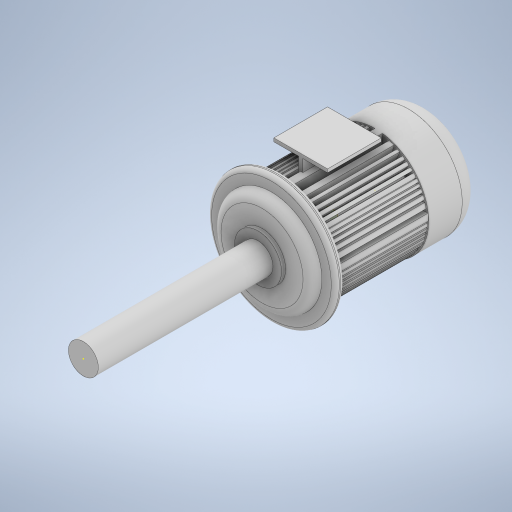
# Autodesk Inventor part: chanti eg
Saved by Autodesk Inventor 2023 (Build 270158000, 158)
## iProperties
Created: 2023-11-02
Part Number: chanti eg
Material: Generic
Document SubType Name: Modeling
Designer: chanti
Density: 1 g/cm^3
Appearance: Default
Author: chanti
Autodesk Inventor part; units mm, degrees
ref_plane "YZ Plane" through (0, 0, 0) normal (1, 0, 0) x (0, 1, 0)
ref_plane "XZ Plane" through (0, 0, 0) normal (0, 1, 0) x (-1, 0, 0)
ref_plane "XY Plane" through (0, 0, 0) normal (0, 0, 1) x (1, 0, 0)
sketch "Sketch1" plane through (0, 0, 0) normal (0, 0, 1) x (1, 0, 0)
  circle A0 centre (0, 0) radius 40
  dimension "d0" = 80
  constraints: 1 centre point, 1 coincident
  measures "d0" diameter of A0
extrude "Extrusion1" add sketch "Sketch1" along normal blind 40
sketch "Sketch2" plane through (0, 0, 40) normal (0, 0, 1) x (1, 0, 0)
  circle A0 centre (0, 0) radius 30
  dimension "d3" = 60
  constraints: 1 centre point, 1 coincident
  measures "d3" diameter of A0
sketch "Sketch3" plane through (0, 0, 40) normal (0, 0, 1) x (1, 0, 0)
  line L0 (-0.020624, 29.697668) -> (-0.020624, 39.999995)
  circle A0 centre (0, 0) radius 40
  line L1 (5.634227, 39.601206) -> (5.191892, 29.470084)
  line L2 (5.191892, 29.470084) -> (-0.020624, 29.697668)
  dimension "d4" = 2.5
  constraints: 6 end point, 2 point on circle, 1 perpendicular, 1 vertical
  measures "d4" angle of L0 L1
extrude "Extrusion2" add sketch "Sketch3" along normal blind 70 contours L0 A0 L1 L2 picked at (2.975845, 32.996997)
sketch "Sketch4" plane through (0, 0, 40) normal (0, 0, 1) x (1, 0, 0)
  circle A0 centre (0, 0) radius 40
  line L0 (0, -40) -> (0, -30.033316)
  line L1 (0, -30.033316) -> (2.293817, -30.033316)
  line L2 (2.293817, -30.033316) -> (2.710552, -40)
  line L3 (2.710552, -40) -> (0, -40)
  point P0 (0, -35.016658)
  dimension "d7" = 2.5
  constraints: 8 end point, 2 perpendicular, 1 midpoint, 1 vertical, 1 vertical alignment, 1 other
  measures "d7" distance from line of point (0, -35.017) L2
extrude "Extrusion3" add sketch "Sketch4" along normal blind 70 contours L0 L1 L2 A0 | A0 L2 L3 picked at (1.065557, -33.352147)
sketch "Sketch5" plane through (0, 0, 40) normal (0, 0, 1) x (1, 0, 0)
  circle A0 centre (0, 0) radius 40
  line L0 (6.760588, -39.424541) -> (5.721207, -29.502254)
  line L1 (5.721207, -29.502254) -> (7.131952, -29.354476)
  line L2 (7.131952, -29.354476) -> (10.234211, -38.207292)
  line L3 (10.234211, -38.207292) -> (6.760588, -39.424541)
  point P0 (8.683082, -33.780884)
  dimension "d10" = 2.5
  constraints: 8 end point, 2 perpendicular, 1 midpoint, 2 other
  measures "d10" distance from line of point (8.683, -33.781) L0
extrude "Extrusion4" add sketch "Sketch5" along normal blind 70 contours L0 L1 L2 L3
sketch "Sketch6" plane through (0, 0, 40) normal (0, 0, 1) x (1, 0, 0)
  line L0 (-11.207509, 27.841165) -> (-12.326876, 38.053227)
  circle A0 centre (0, 0) radius 40
  line L1 (-9.924989, 39.08492) -> (-8.805622, 28.872858)
  line L2 (-8.805622, 28.872858) -> (-11.207509, 27.841165)
  line L3 (-9.924989, 39.08492) -> (-12.326876, 38.053227)
  line L4 (-17.739765, 24.864744) -> (-18.904942, 35.49473)
  line L5 (-18.904942, 35.49473) -> (-21.743257, 32.947196)
  line L6 (-21.743257, 32.947196) -> (-19.480863, 23.302019)
  line L7 (-19.480863, 23.302019) -> (-17.739765, 24.864744)
  point P0 (-20.61206, 28.124608)
  point P1 (-9.365305, 33.978889)
  dimension "d13" = 2.5
  dimension "d14" = 2.5
  constraints: 16 end point, 4 parallel, 2 midpoint, 2 other
  measures "d13" distance from line of L4 point (-20.612, 28.125)
  measures "d14" distance from line of point (-9.365, 33.979) L0
extrude "Extrusion5" add sketch "Sketch6" along normal blind 70 contours L4 L7 L6 L5 A0 | A0 L5 L4
sketch "Sketch7" plane through (0, 0, 40) normal (0, 0, 1) x (1, 0, 0)
  point P0 (0, 0)
sketch "Sketch8" plane through (0, 0, 40) normal (0, 0, 1) x (1, 0, 0)
  line L0 (30.442143, 0) -> (39.650787, 0)
  line L1 (39.650787, 0) -> (39.650787, 5.274002)
  arc A0 (6.760588, -39.424541) -> (5.634227, 39.601206) centre (0, 0) ccw
  line L2 (30.442143, 4.39287) -> (30.442143, 0)
  line L3 (30.442143, 4.39287) -> (39.650787, 5.274002)
  constraints: 8 end point, 1 horizontal, 1 parallel, 1 perpendicular, 1 point on circle
extrude "Extrusion6" add sketch "Sketch8" along normal blind 70
sketch "Sketch9" plane through (0, 0, 40) normal (0, 0, 1) x (1, 0, 0)
  line L0 (10.675749, 37.596929) -> (8.268351, 29.06161)
  line L1 (8.268351, 29.06161) -> (12.000604, 28.008924)
  line L2 (12.000604, 28.008924) -> (14.408001, 36.544243)
  line L3 (14.408001, 36.544243) -> (10.675749, 37.596929)
  point P0 (0, 0)
  constraints: 8 end point, 3 perpendicular
extrude "Extrusion7" add sketch "Sketch9" along normal blind 70
sketch "Sketch10" plane through (0, 0, 40) normal (0, 0, 1) x (1, 0, 0)
  line L0 (13.617247, 27.55159) -> (16.676639, 35.171207)
  line L1 (16.676639, 35.171207) -> (18.671094, 34.300788)
  line L2 (18.671094, 34.300788) -> (15.388296, 26.77867)
  line L3 (15.388296, 26.77867) -> (13.617247, 27.55159)
  point P0 (0, 0)
  constraints: 8 end point, 2 perpendicular
extrude "Extrusion8" add sketch "Sketch10" along normal blind 70
sketch "Sketch11" plane through (0, 0, 40) normal (0, 0, 1) x (1, 0, 0)
  line L0 (16.809785, 25.989212) -> (20.82419, 32.823259)
  line L1 (20.82419, 32.823259) -> (22.496859, 31.15059)
  line L2 (22.496859, 31.15059) -> (18.182558, 25.182829)
  arc A0 (18.182558, 25.182829) -> (16.809785, 25.989212) centre (13.257658, 18.370456) ccw
  point P0 (0, 0)
  constraints: 6 end point, 2 point on circle, 1 centre point, 1 point on line
extrude "Extrusion9" add sketch "Sketch11" along normal blind 70
sketch "Sketch12" plane through (0, 0, 40) normal (0, 0, 1) x (1, 0, 0)
  line L0 (19.103485, 24.559546) -> (23.864166, 30.764478)
  line L1 (23.864166, 30.764478) -> (25.415399, 28.785319)
  line L2 (25.415399, 28.785319) -> (21.03576, 23.077025)
  line L3 (21.03576, 23.077025) -> (19.103485, 24.559546)
  point P0 (0, 0)
  constraints: 8 end point, 1 parallel, 1 perpendicular
extrude "Extrusion10" add sketch "Sketch12" along normal blind 70
sketch "Sketch13" plane through (0, 0, 40) normal (0, 0, 1) x (1, 0, 0)
  line L0 (21.900009, 22.413937) -> (26.279648, 28.122231)
  line L1 (25.415399, 28.785319) -> (21.03576, 23.077025)
  line L2 (26.279648, 28.122231) -> (28.473032, 27.138104)
  line L3 (28.473032, 27.138104) -> (22.406361, 21.139597)
  line L4 (22.406361, 21.139597) -> (21.900009, 22.413937)
  point P0 (0, 0)
  constraints: 8 end point, 1 parallel
extrude "Extrusion11" add sketch "Sketch13" along normal blind 70
sketch "Sketch14" plane through (0, 0, 40) normal (0, 0, 1) x (1, 0, 0)
  line L0 (23.520225, 20.609732) -> (29.267064, 26.194688)
  line L1 (29.267064, 26.194688) -> (30.562126, 23.40221)
  line L2 (30.562126, 23.40221) -> (24.799945, 19.292919)
  arc A0 (24.799945, 19.292919) -> (23.520225, 20.609732) centre (19.850859, 15.763486) ccw
  point P0 (0, 0)
  constraints: 6 end point, 2 point on circle, 1 centre point, 1 point on line
extrude "Extrusion12" add sketch "Sketch14" along normal blind 70
sketch "Sketch15" plane through (0, 0, 40) normal (0, 0, 1) x (1, 0, 0)
  line L0 (24.833565, 18.287479) -> (31.44559, 23.686911)
  line L1 (31.44559, 23.686911) -> (32.648409, 21.733895)
  line L2 (32.648409, 21.733895) -> (25.754817, 16.957789)
  line L3 (25.754817, 16.957789) -> (24.833565, 18.287479)
  point P0 (0, 0)
  constraints: 8 end point, 1 perpendicular
extrude "Extrusion13" add sketch "Sketch15" along normal blind 70
sketch "Sketch16" plane through (0, 0, 40) normal (0, 0, 1) x (1, 0, 0)
  line L0 (25.958317, 16.60202) -> (32.865906, 20.912961)
  line L1 (32.865906, 20.912961) -> (34.102149, 19.635639)
  line L2 (34.102149, 19.635639) -> (26.878556, 15.127485)
  line L3 (26.878556, 15.127485) -> (25.958317, 16.60202)
  point P0 (0, 0)
  constraints: 8 end point, 1 parallel, 1 perpendicular
extrude "Extrusion14" add sketch "Sketch16" along normal blind 70
sketch "Sketch17" plane through (0, 0, 40) normal (0, 0, 1) x (1, 0, 0)
  line L0 (-30.507216, 0) -> (-40, 0)
  circle A0 centre (0, 0) radius 40
  line L1 (-39.358717, 3.146179) -> (-30.507216, 3.146179)
  line L2 (-30.507216, 3.146179) -> (-30.507216, 0)
  line L3 (-39.358717, 3.146179) -> (-40, 0)
  constraints: 8 end point, 2 horizontal, 1 horizontal alignment, 1 perpendicular, 1 other
extrude "Extrusion15" add sketch "Sketch17" along normal blind 70 contours L0 L3 L1 L2
sketch "Sketch18" plane through (0, 0, 40) normal (0, 0, 1) x (1, 0, 0)
  line L0 (-16.678263, 25.896258) -> (-17.403068, 35.509462)
  line L1 (-17.403068, 35.509462) -> (-14.427552, 36.806482)
  line L2 (-14.427552, 36.806482) -> (-14.427552, 27.65105)
  line L3 (-14.427552, 27.65105) -> (-16.678263, 25.896258)
  point P0 (0, 0)
  constraints: 8 end point, 1 vertical
extrude "Extrusion16" add sketch "Sketch18" along normal blind 70
sketch "Sketch19" plane through (0, 0, 40) normal (0, 0, 1) x (1, 0, 0)
  line L0 (-13.42925, 28.250328) -> (-13.42925, 36.714172)
  line L1 (-13.42925, 36.714172) -> (-10.263385, 37.941753)
  line L2 (-10.263385, 37.941753) -> (-10.263385, 28.250328)
  line L3 (-10.263385, 28.250328) -> (-13.42925, 28.250328)
  point P0 (0, 0)
  constraints: 8 end point, 1 parallel, 1 perpendicular, 1 vertical
extrude "Extrusion17" add sketch "Sketch19" along normal blind 70
sketch "Sketch20" plane through (0, 0, 40) normal (0, 0, 1) x (1, 0, 0)
  line L0 (-9.356562, 29.365782) -> (-9.356562, 38.139886)
  arc A0 (-9.356562, 38.139886) -> (-6.989863, 38.774854) centre (-9.356562, 42.868037) ccw
  line L1 (-6.989863, 38.774854) -> (-6.989863, 29.827577)
  line L2 (-6.989863, 29.827577) -> (-9.356562, 29.365782)
  point P0 (0, 0)
  constraints: 6 end point, 2 point on circle, 1 centre point, 1 parallel, 1 point on line, 1 vertical
extrude "Extrusion18" add sketch "Sketch20" along normal blind 70
sketch "Sketch21" plane through (0, 0, 40) normal (0, 0, 1) x (1, 0, 0)
  line L0 (-6.048793, 30.401226) -> (-6.048793, 38.774854)
  line L1 (-6.048793, 38.774854) -> (-3.722851, 38.774854)
  line L2 (-3.722851, 38.774854) -> (-3.722851, 30.401226)
  line L3 (-3.722851, 30.401226) -> (-6.048793, 30.401226)
  point P0 (0, 0)
  constraints: 8 end point, 3 perpendicular, 1 vertical
extrude "Extrusion19" add sketch "Sketch21" along normal blind 70
sketch "Sketch22" plane through (0, 0, 40) normal (0, 0, 1) x (1, 0, 0)
  line L0 (-30.807767, 4.536279) -> (-38.740023, 4.536279)
  line L1 (-38.740023, 4.536279) -> (-38.740023, 6.964521)
  line L2 (-38.740023, 6.964521) -> (-30.807767, 6.964521)
  line L3 (-30.807767, 6.964521) -> (-30.807767, 4.536279)
  point P0 (0, 0)
  constraints: 8 end point, 2 perpendicular, 1 horizontal
extrude "Extrusion20" add sketch "Sketch22" along normal blind 70
sketch "Sketch23" plane through (0, 0, 40) normal (0, 0, 1) x (1, 0, 0)
  line L0 (-29.843538, 7.57041) -> (-38.358924, 8.133928)
  line L1 (-38.358924, 8.133928) -> (-37.607567, 11.76549)
  line L2 (-37.607567, 11.76549) -> (-28.831291, 9.949709)
  line L3 (-28.831291, 9.949709) -> (-29.843538, 7.57041)
  point P0 (0, 0)
  constraints: 8 end point, 1 perpendicular
extrude "Extrusion21" add sketch "Sketch23" along normal blind 70
sketch "Sketch24" plane through (0, 0, 40) normal (0, 0, 1) x (1, 0, 0)
  line L0 (-28.828399, 10.40498) -> (-37.43399, 12.939835)
  line L1 (-37.43399, 12.939835) -> (-36.368382, 15.76531)
  line L2 (-36.368382, 15.76531) -> (-27.743659, 12.512557)
  line L3 (-27.743659, 12.512557) -> (-28.828399, 10.40498)
  point P0 (0, 0)
  constraints: 8 end point, 1 perpendicular
extrude "Extrusion22" add sketch "Sketch24" along normal blind 70
sketch "Sketch25" plane through (0, 0, 40) normal (0, 0, 1) x (1, 0, 0)
  line L0 (-27.43188, 12.826275) -> (-35.76006, 16.83717)
  line L1 (-35.76006, 16.83717) -> (-34.423802, 19.611763)
  line L2 (-34.423802, 19.611763) -> (-26.1568, 15.234327)
  line L3 (-26.1568, 15.234327) -> (-27.43188, 12.826275)
  point P0 (0, 0)
  constraints: 8 end point, 2 perpendicular
extrude "Extrusion23" add sketch "Sketch25" along normal blind 70
sketch "Sketch26" plane through (0, 0, 40) normal (0, 0, 1) x (1, 0, 0)
  line L0 (-26.352336, 15.926773) -> (-33.405662, 20.704831)
  line L1 (-33.405662, 20.704831) -> (-31.807338, 23.064262)
  line L2 (-31.807338, 23.064262) -> (-24.952655, 17.723071)
  line L3 (-24.952655, 17.723071) -> (-26.352336, 15.926773)
  point P0 (0, 0)
  constraints: 8 end point, 1 perpendicular
extrude "Extrusion24" add sketch "Sketch26" along normal blind 70
sketch "Sketch27" plane through (0, 0, 40) normal (0, 0, 1) x (1, 0, 0)
  line L0 (-24.562055, 19.042614) -> (-31.089513, 23.734224)
  line L1 (-31.089513, 23.734224) -> (-29.420556, 26.056251)
  line L2 (-29.420556, 26.056251) -> (-23.527222, 20.059623)
  line L3 (-23.527222, 20.059623) -> (-24.562055, 19.042614)
  point P0 (0, 0)
  constraints: 8 end point, 2 perpendicular
extrude "Extrusion25" add sketch "Sketch27" along normal blind 70
sketch "Sketch28" plane through (0, 0, 40) normal (0, 0, 1) x (1, 0, 0)
  line L0 (-22.488904, 21.229021) -> (-27.687491, 27.759464)
  line L1 (-27.687491, 27.759464) -> (-25.054931, 29.855125)
  line L2 (-25.054931, 29.855125) -> (-20.019904, 23.057937)
  line L3 (-20.019904, 23.057937) -> (-22.488904, 21.229021)
  point P0 (0, 0)
  constraints: 8 end point, 2 perpendicular
extrude "Extrusion26" add sketch "Sketch28" along normal blind 70
sketch "Sketch29" plane through (0, 0, 40) normal (0, 0, 1) x (1, 0, 0)
  line L0 (-21.429697, 25.910274) -> (-24.881325, 30.391969)
  line L1 (-24.881325, 30.391969) -> (-22.502598, 32.223972)
  line L2 (-22.502598, 32.223972) -> (-20.741788, 26.440074)
  line L3 (-20.741788, 26.440074) -> (-21.429697, 25.910274)
  point P0 (0, 0)
  constraints: 8 end point, 1 parallel, 1 perpendicular
extrude "Extrusion27" add sketch "Sketch29" along normal blind 70
sketch "Sketch30" plane through (0, 0, 40) normal (0, 0, 1) x (1, 0, 0)
  line L0 (27.344535, 14.453695) -> (34.492836, 18.448334)
  line L1 (34.492836, 18.448334) -> (35.608985, 16.451014)
  line L2 (35.608985, 16.451014) -> (28.460684, 12.456376)
  line L3 (28.460684, 12.456376) -> (27.344535, 14.453695)
  point P0 (0, 0)
  constraints: 8 end point, 2 perpendicular
extrude "Extrusion28" add sketch "Sketch30" along normal blind 70
sketch "Sketch31" plane through (0, 0, 40) normal (0, 0, 1) x (1, 0, 0)
  line L0 (28.700168, 11.511497) -> (36.106904, 15.318311)
  line L1 (36.106904, 15.318311) -> (36.975851, 12.504579)
  line L2 (36.975851, 12.504579) -> (29.393297, 10.162908)
  line L3 (29.393297, 10.162908) -> (28.938925, 11.63421)
  point P0 (0, 0)
  constraints: 8 end point, 1 point on line
extrude "Extrusion29" add sketch "Sketch31" along normal blind 70
sketch "Sketch32" plane through (0, 0, 40) normal (0, 0, 1) x (1, 0, 0)
  line L0 (30.068133, 8.998603) -> (37.178617, 10.945522)
  line L1 (37.178617, 10.945522) -> (38.168632, 7.329814)
  arc A0 (30.068133, 6.12055) -> (38.168632, 7.329814) centre (29.064478, 40.579769) ccw
  line L2 (30.068133, 6.12055) -> (30.068133, 8.998603)
  point P0 (0, 0)
  constraints: 6 end point, 2 point on circle, 1 centre point, 1 perpendicular, 1 point on line, 1 vertical
extrude "Extrusion30" add sketch "Sketch32" along normal blind 70
sketch "Sketch33" plane through (0, 0, 40) normal (0, 0, 1) x (1, 0, 0)
  line L0 (-30.266675, -1.157847) -> (-39.598353, -1.157847)
  line L1 (-39.598353, -1.157847) -> (-39.598353, -4.07562)
  line L2 (-39.598353, -4.07562) -> (-30.104011, -3.380912)
  line L3 (-30.104011, -3.380912) -> (-30.266675, -1.157847)
  point P0 (0, 0)
  constraints: 8 end point, 2 perpendicular, 1 horizontal
extrude "Extrusion31" add sketch "Sketch33" along normal blind 70
sketch "Sketch34" plane through (0, 0, 40) normal (0, 0, 1) x (1, 0, 0)
  line L0 (-30.061013, -4.317752) -> (-39.227843, -5.511349)
  line L1 (-39.227843, -5.511349) -> (-38.880572, -8.178387)
  arc A0 (-38.880572, -8.178387) -> (-30.061013, -6.46218) centre (-48.136658, 62.90836) ccw
  line L2 (-30.061013, -4.317752) -> (-30.061013, -6.46218)
  point P0 (0, 0)
  constraints: 6 end point, 2 point on circle, 1 centre point, 1 perpendicular, 1 point on line, 1 vertical
extrude "Extrusion32" add sketch "Sketch34" along normal blind 70
sketch "Sketch35" plane through (0, 0, 40) normal (0, 0, 1) x (1, 0, 0)
  line L0 (-29.717279, -7.227233) -> (-38.170745, -9.791768)
  line L1 (-38.170745, -9.791768) -> (-37.356249, -12.47659)
  line L2 (-37.356249, -12.47659) -> (-28.946165, -9.216458)
  line L3 (-28.946165, -9.216458) -> (-29.717279, -7.227233)
  point P0 (0, 0)
  constraints: 8 end point, 2 perpendicular
extrude "Extrusion33" add sketch "Sketch35" along normal blind 70
sketch "Sketch36" plane through (0, 0, 40) normal (0, 0, 1) x (1, 0, 0)
  line L0 (-28.946165, -10.142735) -> (-37.190033, -13.338392)
  line L1 (-37.190033, -13.338392) -> (-36.18894, -15.92092)
  line L2 (-36.18894, -15.92092) -> (-27.788318, -11.740564)
  arc A0 (-27.788318, -11.740564) -> (-28.946165, -10.142735) centre (-33.155513, -14.411412) ccw
  point P0 (0, 0)
  constraints: 6 end point, 2 point on circle, 1 centre point, 1 perpendicular, 1 point on line
extrude "Extrusion34" add sketch "Sketch36" along normal blind 70
sketch "Sketch37" plane through (0, 0, 40) normal (0, 0, 1) x (1, 0, 0)
  line L0 (-27.990789, -13.014096) -> (-35.140486, -17.205298)
  line L1 (-35.140486, -17.205298) -> (-33.791588, -19.506358)
  line L2 (-33.791588, -19.506358) -> (-26.788448, -14.805164)
  line L3 (-26.788448, -14.805164) -> (-27.990789, -13.014096)
  point P0 (0, 0)
  constraints: 8 end point, 2 perpendicular
extrude "Extrusion35" add sketch "Sketch37" along normal blind 70
sketch "Sketch38" plane through (0, 0, 40) normal (0, 0, 1) x (1, 0, 0)
  line L0 (-33.280962, -20.63459) -> (-31.086051, -23.444076)
  line L1 (-31.086051, -23.444076) -> (-24.586239, -18.366098)
  line L2 (-24.586239, -18.366098) -> (-26.78115, -15.556612)
  line L3 (-26.78115, -15.556612) -> (-33.280962, -20.63459)
  point P0 (0, 0)
  constraints: 8 end point, 3 perpendicular
extrude "Extrusion36" add sketch "Sketch38" along normal blind 70
sketch "Sketch39" plane through (0, 0, 40) normal (0, 0, 1) x (1, 0, 0)
  line L0 (-24.005075, -19.41135) -> (-30.445791, -24.69604)
  line L1 (-30.445791, -24.69604) -> (-29.223572, -26.71105)
  arc A0 (-29.223572, -26.71105) -> (-22.782991, -21.426138) centre (-44.496403, -1.531518) ccw
  line L2 (-22.782991, -21.426138) -> (-24.005075, -19.41135)
  point P0 (0, 0)
  constraints: 6 end point, 2 point on circle, 1 centre point, 1 parallel, 1 point on line
extrude "Extrusion37" add sketch "Sketch39" along normal blind 70
sketch "Sketch40" plane through (0, 0, 40) normal (0, 0, 1) x (1, 0, 0)
  line L0 (-22.120067, -21.795) -> (-28.28323, -27.419896)
  line L1 (-28.28323, -27.419896) -> (-26.743166, -29.107335)
  line L2 (-26.743166, -29.107335) -> (-20.973524, -22.852626)
  line L3 (-20.973524, -22.852626) -> (-22.120067, -21.795)
  point P0 (0, 0)
  constraints: 8 end point, 2 perpendicular
extrude "Extrusion38" add sketch "Sketch40" along normal blind 70
sketch "Sketch41" plane through (0, 0, 40) normal (0, 0, 1) x (1, 0, 0)
  line L0 (-25.692263, -29.66427) -> (-20.058062, -23.576822)
  line L1 (-20.058062, -23.576822) -> (-18.197513, -24.508106)
  line L2 (-18.197513, -24.508106) -> (-23.876013, -31.20445)
  line L3 (-23.876013, -31.20445) -> (-25.692263, -29.66427)
  point P0 (0, 0)
  constraints: 8 end point, 1 perpendicular
extrude "Extrusion39" add sketch "Sketch41" along normal blind 70
sketch "Sketch42" plane through (0, 0, 40) normal (0, 0, 1) x (1, 0, 0)
  line L0 (-17.24899, -26.468279) -> (-23.061331, -32.682947)
  circle A0 centre (0, 0) radius 40
  line L1 (-20.061293, -32.58259) -> (-15.698793, -27.918119)
  line L2 (-15.698793, -27.918119) -> (-17.24899, -26.468279)
  arc A1 (-23.061331, -32.682947) -> (-20.061293, -32.58259) centre (-21.611491, -31.132749) ccw
  constraints: 6 end point, 2 point on circle, 1 centre point, 1 parallel, 1 perpendicular, 1 point on line, 1 tangent, 2 other
extrude "Extrusion40" add sketch "Sketch42" along normal blind 70 contours L2 L1 A1 A0 L0 | A0 A1 picked at (-20.123871, -30.577939)
sketch "Sketch43" plane through (0, 0, 40) normal (0, 0, 1) x (1, 0, 0)
  line L0 (-1.756912, -39.43757) -> (-1.756912, -30.685514)
  line L1 (-1.756912, -30.685514) -> (-4.39146, -30.149674)
  line L2 (-4.39146, -30.149674) -> (-4.39146, -39.080344)
  line L3 (-4.39146, -39.080344) -> (-1.756912, -39.080344)
  point P0 (0, 0)
  constraints: 8 end point, 1 parallel, 1 point on line, 1 vertical
extrude "Extrusion41" add sketch "Sketch43" along normal blind 70
sketch "Sketch44" plane through (0, 0, 40) normal (0, 0, 1) x (1, 0, 0)
  line L0 (-20.211042, -34.096481) -> (-14.438552, -27.13989)
  line L1 (-14.438552, -27.13989) -> (-12.573594, -27.918119)
  line L2 (-12.573594, -27.918119) -> (-18.724128, -35.330302)
  line L3 (-18.724128, -35.330302) -> (-20.211042, -34.096481)
  point P0 (0, 0)
  constraints: 8 end point, 1 parallel, 1 perpendicular
extrude "Extrusion42" add sketch "Sketch44" along normal blind 70
sketch "Sketch45" plane through (0, 0, 40) normal (0, 0, 1) x (1, 0, 0)
  line L0 (-17.136687, -35.73742) -> (-12.260235, -28.046957)
  line L1 (-12.260235, -28.046957) -> (-10.634751, -28.361566)
  line L2 (-10.634751, -28.361566) -> (-15.550493, -36.743211)
  arc A0 (-17.136687, -35.73742) -> (-15.550493, -36.743211) centre (-1.850137, -13.383257) ccw
  point P0 (0, 0)
  constraints: 6 end point, 2 point on circle, 1 centre point, 1 point on line
extrude "Extrusion43" add sketch "Sketch45" along normal blind 70
sketch "Sketch46" plane through (0, 0, 40) normal (0, 0, 1) x (1, 0, 0)
  line L0 (-14.118893, -36.870331) -> (-9.496341, -28.988593)
  line L1 (-15.550493, -36.743211) -> (-10.634751, -28.361566)
  line L2 (-9.496341, -28.988593) -> (-7.270064, -29.71956)
  line L3 (-7.270064, -29.71956) -> (-11.892617, -37.601298)
  line L4 (-11.892617, -37.601298) -> (-14.118893, -36.870331)
  point P0 (0, 0)
  constraints: 8 end point, 3 parallel
extrude "Extrusion44" add sketch "Sketch46" along normal blind 70
sketch "Sketch47" plane through (0, 0, 40) normal (0, 0, 1) x (1, 0, 0)
  line L0 (-10.917292, -37.923259) -> (-6.759072, -29.859197)
  line L1 (-6.759072, -29.859197) -> (-4.992429, -30.111574)
  arc A0 (-6.759072, -38.187655) -> (-4.992429, -30.111574) centre (-60.745603, -22.146835) ccw
  line L2 (-6.759072, -38.187655) -> (-10.917292, -37.923259)
  point P0 (0, 0)
  constraints: 6 end point, 2 point on circle, 1 centre point, 1 point on line
extrude "Extrusion45" add sketch "Sketch47" along normal blind 70
sketch "Sketch48" plane through (0, 0, 40) normal (0, 0, 1) x (1, 0, 0)
  line L0 (30.316609, -1.654587) -> (39.143968, -1.236449)
  line L1 (39.143968, -1.236449) -> (39.264633, -3.783821)
  line L2 (39.264633, -3.783821) -> (30.41724, -3.783821)
  arc A0 (30.41724, -3.783821) -> (30.316609, -1.654587) centre (7.840965, -3.783821) ccw
  point P0 (0, 0)
  constraints: 6 end point, 2 point on circle, 1 centre point, 1 horizontal, 1 perpendicular, 1 point on line
extrude "Extrusion46" add sketch "Sketch48" along normal blind 70
sketch "Sketch49" plane through (0, 0, 40) normal (0, 0, 1) x (1, 0, 0)
  line L0 (29.957256, -4.842652) -> (39.098479, -4.842652)
  line L1 (39.098479, -4.842652) -> (38.445535, -7.213872)
  line L2 (38.445535, -7.213872) -> (29.957256, -6.732755)
  arc A0 (29.957256, -6.732755) -> (29.957256, -4.842652) centre (13.283851, -5.787703) ccw
  point P0 (0, 0)
  constraints: 6 end point, 2 point on circle, 1 centre point, 1 horizontal, 1 point on line
extrude "Extrusion47" add sketch "Sketch49" along normal blind 70
sketch "Sketch50" plane through (0, 0, 40) normal (0, 0, 1) x (1, 0, 0)
  line L0 (29.448185, -8.271081) -> (38.253673, -8.490532)
  line L1 (38.253673, -8.490532) -> (37.513025, -10.904498)
  line L2 (37.513025, -10.904498) -> (28.652674, -10.273575)
  arc A0 (29.448185, -8.271081) -> (28.652674, -10.273575) centre (32.208108, -10.526748) ccw
  point P0 (0, 0)
  constraints: 6 end point, 2 point on circle, 1 centre point, 1 point on line
extrude "Extrusion48" add sketch "Sketch50" along normal blind 70
sketch "Sketch51" plane through (0, 0, 40) normal (0, 0, 1) x (1, 0, 0)
  line L0 (28.3844, -11.035723) -> (37.486925, -11.887519)
  line L1 (37.486925, -11.887519) -> (36.501514, -14.626627)
  line L2 (36.501514, -14.626627) -> (27.482498, -12.672507)
  arc A0 (28.3844, -11.035723) -> (27.482498, -12.672507) centre (30.673356, -13.36386) ccw
  point P0 (0, 0)
  constraints: 6 end point, 2 point on circle, 1 centre point, 1 point on line
extrude "Extrusion49" add sketch "Sketch51" along normal blind 70
sketch "Sketch52" plane through (0, 0, 40) normal (0, 0, 1) x (1, 0, 0)
  line L0 (27.200819, -13.347504) -> (36.147284, -15.713404)
  line L1 (36.147284, -15.713404) -> (35.306937, -17.54924)
  line L2 (35.306937, -17.54924) -> (26.463899, -14.743773)
  arc A0 (27.200819, -13.347504) -> (26.463899, -14.743773) centre (30.703747, -16.088871) ccw
  point P0 (0, 0)
  constraints: 6 end point, 2 point on circle, 1 centre point, 1 point on line
extrude "Extrusion50" add sketch "Sketch52" along normal blind 70
sketch "Sketch53" plane through (0, 0, 40) normal (0, 0, 1) x (1, 0, 0)
  line L0 (10.234211, -29.354476) -> (12.997182, -37.239075)
  line L1 (7.131952, -29.354476) -> (10.234211, -38.207292)
  line L2 (12.997182, -37.239075) -> (14.783813, -36.612993)
  line L3 (14.783813, -36.612993) -> (12.020842, -28.728393)
  line L4 (12.020842, -28.728393) -> (10.234211, -29.354476)
  point P0 (0, 0)
  constraints: 8 end point, 3 perpendicular, 1 parallel
extrude "Extrusion51" add sketch "Sketch53" along normal blind 70
sketch "Sketch54" plane through (0, 0, 40) normal (0, 0, 1) x (1, 0, 0)
  line L0 (12.795702, -28.033498) -> (15.696401, -36.340045)
  arc A0 (15.696401, -36.340045) -> (19.693506, -33.265922) centre (13.05109, -28.764836) ccw
  line L1 (19.693506, -33.265922) -> (14.701135, -27.368108)
  line L2 (14.701135, -27.368108) -> (13.05109, -28.764836)
  point P0 (0, 0)
  constraints: 6 end point, 2 point on circle, 1 centre point, 1 perpendicular, 1 point on line
extrude "Extrusion52" add sketch "Sketch54" along normal blind 70
sketch "Sketch55" plane through (0, 0, 40) normal (0, 0, 1) x (1, 0, 0)
  line L0 (15.689361, -26.655563) -> (20.865009, -33.088155)
  line L1 (20.865009, -33.088155) -> (23.600709, -31.350616)
  arc A0 (23.600709, -31.350616) -> (17.681196, -25.052938) centre (4.143535, -43.708551) ccw
  line L2 (15.689361, -26.655563) -> (17.681196, -25.052938)
  point P0 (0, 0)
  constraints: 6 end point, 2 point on circle, 1 centre point, 1 point on line
extrude "Extrusion53" add sketch "Sketch55" along normal blind 70
sketch "Sketch56" plane through (0, 0, 40) normal (0, 0, 1) x (1, 0, 0)
  line L0 (26.566601, -15.241881) -> (34.519037, -17.723492)
  arc A0 (33.478236, -19.471261) -> (34.519037, -17.723492) centre (30.342634, -16.420218) ccw
  line L1 (33.478236, -19.471261) -> (25.977237, -17.130524)
  line L2 (25.977237, -17.130524) -> (26.566601, -15.241881)
  point P0 (0, 0)
  constraints: 6 end point, 2 point on circle, 1 centre point, 1 perpendicular, 1 point on line
extrude "Extrusion54" add sketch "Sketch56" along normal blind 70
sketch "Sketch57" plane through (0, 0, 40) normal (0, 0, 1) x (1, 0, 0)
  line L0 (18.959873, -24.405106) -> (24.979237, -30.540228)
  line L1 (24.979237, -30.540228) -> (27.296554, -28.266634)
  arc A0 (27.296554, -28.266634) -> (22.702683, -24.405106) centre (4.932593, -50.208634) ccw
  line L2 (22.702683, -24.405106) -> (20.86692, -22.534041)
  line L3 (20.86692, -22.534041) -> (18.959873, -24.405106)
  point P0 (0, 0)
  constraints: 8 end point, 3 perpendicular, 2 point on circle, 1 centre point, 1 point on line
extrude "Extrusion55" add sketch "Sketch57" along normal blind 70
sketch "Sketch58" plane through (0, 0, 40) normal (0, 0, 1) x (1, 0, 0)
  line L0 (21.638249, -22.04791) -> (27.918374, -27.630243)
  line L1 (27.918374, -27.630243) -> (29.727736, -25.59471)
  line L2 (29.727736, -25.59471) -> (23.447611, -20.012377)
  line L3 (23.447611, -20.012377) -> (21.638249, -22.04791)
  point P0 (0, 0)
  constraints: 8 end point, 1 perpendicular
extrude "Extrusion56" add sketch "Sketch58" along normal blind 70
sketch "Sketch59" plane through (0, 0, 40) normal (0, 0, 1) x (1, 0, 0)
  line L0 (24.054237, -19.44184) -> (25.708978, -17.683677)
  line L1 (25.708978, -17.683677) -> (32.01768, -21.9929)
  line L2 (32.01768, -21.9929) -> (30.292903, -24.517973)
  arc A0 (24.054237, -19.44184) -> (30.292903, -24.517973) centre (57.409132, 15.180186) ccw
  point P0 (0, 0)
  constraints: 6 end point, 2 point on circle, 1 centre point, 1 point on line
extrude "Extrusion57" add sketch "Sketch59" along normal blind 70
sketch "Sketch60" plane through (0, 0, 40) normal (0, 0, 1) x (1, 0, 0)
  line L0 (3.880277, -39.73052) -> (3.491265, -30.426831)
  line L1 (2.293817, -30.033316) -> (2.706718, -39.908316)
  line L2 (3.491265, -30.426831) -> (4.659828, -30.37797)
  line L3 (4.659828, -30.37797) -> (5.048775, -39.680094)
  circle A0 centre (0, 0) radius 40
  line L4 (3.880277, -39.73052) -> (3.878169, -39.680094)
  line L5 (3.878169, -39.680094) -> (5.048775, -39.680094)
  constraints: 10 end point, 1 horizontal, 1 parallel, 1 perpendicular, 1 point on circle, 1 point on line
extrude "Extrusion58" add sketch "Sketch60" along normal blind 70 contours L0 L2 L3 L5
extrude "Extrusion59" add sketch "Sketch2" along normal blind 70
sketch "Sketch61" plane through (0, 0, 110) normal (0, 0, 1) x (1, 0, 0)
  circle A0 centre (0, 0) radius 47.5
  dimension "d125" = 95
  constraints: 1 centre point, 1 coincident
  measures "d125" diameter of A0
extrude "Extrusion60" add sketch "Sketch61" along normal blind 7
sketch "Sketch62" plane through (0, 0, 117) normal (0, 0, 1) x (1, 0, 0)
  circle A0 centre (0, 0) radius 37.5
  dimension "d128" = 75
  constraints: 1 centre point, 1 coincident
  measures "d128" diameter of A0
extrude "Extrusion61" add sketch "Sketch62" along normal blind 7
fillet "Fillet1" radius 7 1 edges at (-37.5, 0, 124)
fillet "Fillet2" radius 3 1 edges at (-47.5, 0, 117)
fillet "Fillet3" radius 3 1 edges at (-47.5, 0, 110)
sketch "Sketch63" plane through (0, 0, 124) normal (0, 0, 1) x (1, 0, 0)
  circle A0 centre (0, 0) radius 17.5
  dimension "d134" = 35
  constraints: 1 centre point, 1 coincident
  measures "d134" diameter of A0
extrude "Extrusion62" add sketch "Sketch63" along normal blind 3
sketch "Sketch64" plane through (0, 0, 127) normal (0, 0, 1) x (1, 0, 0)
  circle A0 centre (0, 0) radius 17.5 projected
  circle A1 centre (0, 0) radius 11.1125
  dimension "d137" = 22.225
  constraints: 1 centre point, 1 coincident
  measures "d137" diameter of A1
extrude "Extrusion63" add sketch "Sketch64" along normal blind 130 contours A1
fillet "Fillet4" radius 15 1 edges at (-40, 0, 0)
sketch "Sketch65" plane through (0, -40, 40) normal (-1, 0, 0) x (0, 0, 1)
  line L0 (0, 0.575459) -> (70, 0.575459)
  line L1 (54.331463, 0.575459) -> (54.331463, -4.728991)
  line L2 (0, 0) -> (70, 0)
  line L3 (54.331463, -4.728991) -> (37.595249, -4.728991)
  line L4 (37.595249, -4.728991) -> (37.595249, 0.575459)
  line L5 (37.595249, 0.575459) -> (54.331463, 0.575459)
  point P0 (-40, 40)
  point P1 (54.331463, 0)
  point P2 (37.595249, 0)
  dimension "d141" = 5.30445
  constraints: 8 end point, 3 perpendicular, 1 point on line
  measures "d141" distance between parallel lines of L3 L0
extrude "Extrusion64" add sketch "Sketch65" along normal mid plane 20 contours L2 L1 L3 L4
sketch "Sketch66" plane through (5.195239, 29.546734, 110) normal (0.9990482, -0.0436194, 0) x (0, 0, -1)
  line L0 (32.404751, -70.143348) -> (32.404751, -74.867838)
  line L1 (32.404751, -74.262659) -> (44.873424, -74.262659)
  line L2 (44.873424, -74.262659) -> (44.873424, -81.262659)
  line L3 (44.873424, -81.262659) -> (10.098337, -81.262659)
  line L4 (10.098337, -81.262659) -> (10.098337, -74.262659)
  line L5 (10.098337, -74.262659) -> (16.133683, -74.262659)
  line L6 (16.133683, -74.262659) -> (32.404751, -74.262659)
  point P0 (110, -29.745225)
  point P1 (13.11601, -74.262659)
  dimension "d144" = 7
  constraints: 12 end point, 3 point on line, 2 perpendicular, 1 collinear, 1 horizontal, 1 midpoint
  measures "d144" distance from line of L3 point (13.116, -74.263)
extrude "Extrusion65" add sketch "Sketch66" along normal mid plane 40
sketch "Sketch67" plane through (0, 0, 257) normal (0, 0, 1) x (1, 0, 0)
  point P0 (0, 0)
sketch "Sketch68" plane through (0, 0, 257) normal (0, 0, 1) x (1, 0, 0)
  point P0 (0, 0)
sketch "Sketch69" plane through (25.176203, 28.674346, 110) normal (0.9990482, -0.0436194, 0) x (0, 0, -1)
  line L0 (10.098337, -74.262659) -> (44.873424, -74.262659)
  line L1 (44.873424, -81.262659) -> (10.098337, -81.262659)
  line L2 (10.098337, -74.262659) -> (44.873424, -74.262659)
  line L3 (44.873424, -74.262659) -> (44.873424, -81.262659)
  line L4 (44.873424, -81.262659) -> (10.098337, -81.262659)
  line L5 (10.098337, -81.262659) -> (10.098337, -74.262659)
  point P0 (110, -29.745225)
  point P1 (10.098337, -81.262659)
  constraints: 8 end point, 2 parallel, 1 horizontal, 1 perpendicular
extrude "Extrusion66" cut sketch "Sketch69" against normal blind 71.9125
sketch "Sketch70" plane through (-10, -40, 40) normal (-1, 0, 0) x (0, 0, 1)
  line L0 (54.331463, 0) -> (54.331463, -4.728991)
  line L1 (54.331463, 0) -> (37.595249, 0)
  line L2 (54.331463, -4.728991) -> (37.595249, -4.728991)
  line L3 (37.595249, -4.728991) -> (37.595249, 0)
  line L4 (37.595249, 0) -> (54.331463, 0)
  line L5 (54.331463, 0) -> (54.331463, -4.728991)
  point P0 (-40, 40)
  constraints: 8 end point, 2 parallel, 1 horizontal, 1 perpendicular
extrude "Extrusion67" cut sketch "Sketch70" against normal blind 71.9125
ref_plane "Work Plane1" through (0, 0, 95.25) normal (0, 0, -1) x (-1, 0, 0)
sketch "Sketch71" plane through (0, 0, 95.25) normal (0, 0, -1) x (-1, 0, 0)
  circle A0 centre (0, 0) radius 11.1125 projected
  line L0 (0, 0) -> (0, 49)
  line L1 (0, 49) -> (20, 49)
  line L2 (0, 49) -> (0, 51.517)
  line L3 (0, 51.517) -> (20, 51.517)
  line L4 (20, 51.517) -> (20, 49)
  line L5 (0, 49) -> (-20, 49)
  line L6 (0, 51.517) -> (-20, 51.517)
  line L7 (-20, 51.517) -> (-20, 49)
  line L8 (0, 51.517) -> (1.5875, 51.517)
  line L9 (1.5875, 51.517) -> (1.5875, 25.4)
  line L10 (1.5875, 25.4) -> (0, 25.4)
  line L11 (0, 25.4) -> (0, 51.517)
  line L12 (-1.5875, 51.517) -> (-1.5875, 25.4)
  line L13 (-1.5875, 25.4) -> (0, 25.4)
  point P0 (-1.5875, 49)
  point P1 (1.5875, 49)
  dimension "d152" = 49
  dimension "d153" = 2.517
  dimension "d154" = 180
  dimension "d155" = 20
  constraints: 28 end point, 4 symmetric about line, 3 horizontal, 2 parallel, 2 perpendicular, 1 vertical
  measures "d152" distance of L0.start L0.end
  measures "d153" distance of L0.end L2.end
  measures "d154" angle of L6 L3
  measures "d155" distance of L2.end L3.end
extrude "Extrusion68" add sketch "Sketch71" along normal blind 40 contours L13 L12 L5 L0 | L0 L1 L9 L10 | L2 L3 L9 L1 | L5 L12 L6 L2 | L9 L3 L4 L1 | L5 L7 L6 L12
body "Solid1"
